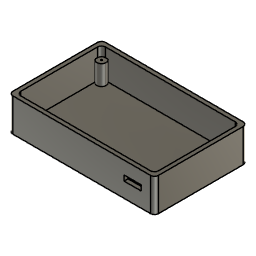
fall_detction_case (Autodesk Fusion 360 design; units mm, degrees)
part number: 2025-06-07-18-41-23-905
Autodesk Fusion 360 part; units mm, degrees
sketch "bottom case" plane through (0, 0, 0) normal (0, 0, 1) x (1, 0, 0)
  line L0 (0, 0) -> (110, 0)
  line L1 (110, 0) -> (110, 70)
  line L2 (110, 70) -> (0, 70)
  line L3 (0, 70) -> (0, 0)
  dimension "d1" = 110
  dimension "d2" = 70
  constraint horizontal L0
  constraint vertical L1
  constraint horizontal L2
  constraint vertical L3
  constraint coincident L0.start L3.end
  measures "d1" distance of L0.start L0.end
  measures "d2" distance of L0.start L2.end
extrude "Extrude1" add sketch "bottom case" along normal blind 25
shell "Shell1" thickness 3 removed faces 1 at (36.6667, 23.3333, 25)
fillet "Fillet3" radius 3 8 edges at (110, 0, 12.5) (107, 3, 14) (107, 67, 14) (110, 70, 12.5) (3, 3, 14) (0, 0, 12.5) (3, 67, 14) (0, 70, 12.5)
cylinder "CylinderPrimitive1" add diameter 7 height 15 placed x (1, 0, 0) y (0, 1, 0) z (0, 0, 1) at (6, 64, 3)
cylinder "CylinderPrimitive2" add diameter 7 height 15 placed x (1, 0, 0) y (0, 1, 0) z (0, 0, 1) at (104, 64, 3)
cylinder "CylinderPrimitive3" add diameter 7 height 15 placed x (1, 0, 0) y (0, 1, 0) z (0, 0, 1) at (6, 6, 3)
cylinder "CylinderPrimitive4" add diameter 7 height 15 placed x (1, 0, 0) y (0, 1, 0) z (0, 0, 1) at (104, 6, 3)
cylinder "CylinderPrimitive5" cut diameter 1.5 height -10 placed x (1, 0, 0) y (0, 1, 0) z (0, 0, 1) at (6, 64, 18)
cylinder "CylinderPrimitive6" cut diameter 1.5 height -10 placed x (1, 0, 0) y (0, 1, 0) z (0, 0, 1) at (104, 64, 18)
cylinder "CylinderPrimitive7" cut diameter 1.5 height -10 placed x (1, 0, 0) y (0, 1, 0) z (0, 0, 1) at (6, 6, 18)
cylinder "CylinderPrimitive8" cut diameter 1.5 height -10 placed x (1, 0, 0) y (0, 1, 0) z (0, 0, 1) at (104, 6, 18)
sketch "charger hole" plane through (0, 0, 0) normal (0, -1, 0) x (1, 0, 0)
  line L0 (3, 25) -> (3, 0)
  line L1 (3, 0) -> (107, 0)
  line L2 (107, 0) -> (107, 25)
  line L3 (107, 25) -> (3, 25)
  line L4 (86.9871, 15.2701) -> (99.9871, 15.2701)
  line L5 (99.9871, 15.2701) -> (99.9871, 11.2701)
  line L6 (99.9871, 11.2701) -> (86.9871, 11.2701)
  line L7 (86.9871, 11.2701) -> (86.9871, 15.2701)
  dimension "d53" = 13
  dimension "d54" = 4
  constraint horizontal L4
  constraint vertical L5
  constraint horizontal L6
  constraint vertical L7
  measures "d53" distance of L4.start L4.end
  measures "d54" distance of L4.start L6.end
extrude "Extrude3" cut sketch "charger hole" against normal blind 3 contours L4 L5 L6 L7
thread "Thread1" "ISO Metric profile 1.4 M1.4x0.3 M1.4x0.3 6H" major diameter 1.4544 minor diameter 1.221 pitch 0.3 angle 60 resizes the face on face at (6.4378, 64.609, 14.6667)
thread "Thread2" "ISO Metric profile 1.4 M1.4x0.3 M1.4x0.3 6H" major diameter 1.4544 minor diameter 1.221 pitch 0.3 angle 60 resizes the face on face at (6.7491, 5.9626, 11.3333)
thread "Thread3" "ISO Metric profile 1.4 M1.4x0.3 M1.4x0.3 6H" major diameter 1.4544 minor diameter 1.221 pitch 0.3 angle 60 resizes the face on face at (104.4069, 64.63, 11.3333)
thread "Thread4" "ISO Metric profile 1.4 M1.4x0.3 M1.4x0.3 6H" major diameter 1.4544 minor diameter 1.221 pitch 0.3 angle 60 resizes the face on face at (104.3085, 5.3164, 14.6667)
named bodies: "bottom cover"
